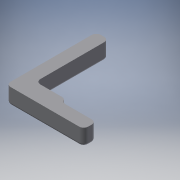
# Autodesk Inventor part: Stand_Vorne
Saved by Autodesk Inventor 2018 (Build 220112000, 112)
## iProperties
Created: 2017-12-09
Part Number: Stand_Vorne
Material: Generisch
Document SubType Name: Modeling
Designer: aXe
Density: 1 g/cm^3
Appearance: Vorgabe
Author: aXe
Autodesk Inventor part; units mm, degrees
ref_plane "YZ Plane" through (0, 0, 0) normal (1, 0, 0) x (0, 1, 0)
ref_plane "XZ Plane" through (0, 0, 0) normal (0, 1, 0) x (-1, 0, 0)
ref_plane "XY Plane" through (0, 0, 0) normal (0, 0, 1) x (1, 0, 0)
sketch "Skizze1" plane through (0, 0, 0) normal (0, 0, 1) x (1, 0, 0)
  line L0 (-2, -29) -> (-2, -31) construction
  line L1 (0, -31) -> (-2, -31) construction
  line L2 (-2, -29) -> (0, -29) construction
  line L3 (0, -31) -> (26.4999, -31) construction
  line L4 (28.4999, -31) -> (26.4999, -31) construction
  line L5 (26.4999, -29) -> (28.4999, -29) construction
  line L6 (28.4999, -31) -> (28.4999, -29) construction
  line L7 (26.4999, -29) -> (0, -29) construction
  line L8 (13, -27) -> (13, -29) construction
  line L9 (13, -27) -> (2, -27) construction
  arc A0 (0, -25) -> (2, -27) centre (2, -25) ccw construction
  arc A1 (-2, -25) -> (2, -29) centre (2, -25) ccw construction
  line L10 (-2, 0) -> (-2, -25) construction
  line L11 (0, -25) -> (0, 0) construction
  line L12 (-2, 0) -> (-2, 5) construction
  line L13 (0, 5) -> (0, 0) construction
  line L14 (0, 5) -> (-2, 5) construction
  line L15 (28.4999, -31) -> (-2, -31) construction
  line L16 (-2, -31) -> (-2, 5) construction
  line L17 (-2, 5) -> (0, 5) construction
  line L18 (0, 5) -> (0, -25) construction
  arc A2 (0, -25) -> (2, -27) centre (2, -25) ccw construction
  line L19 (2, -27) -> (13, -27) construction
  line L20 (13, -27) -> (13, -29) construction
  line L21 (13, -29) -> (28.4999, -29) construction
  line L22 (28.4999, -31) -> (28.4999, -29) construction
  line L23 (-2.25, 5.25) -> (-2.25, -31.25)
  line L24 (-2.25, -31.25) -> (28.7499, -31.25)
  line L25 (28.7499, -31.25) -> (28.7499, -28.75)
  line L26 (28.7499, -28.75) -> (13.25, -28.75)
  line L27 (13.25, -28.75) -> (13.25, -26.75)
  line L28 (13.25, -26.75) -> (2, -26.75)
  arc A3 (0.25, -25) -> (2, -26.75) centre (2, -25) ccw
  line L29 (0.25, -25) -> (0.25, 5.25)
  line L30 (0.25, 5.25) -> (-2.25, 5.25)
  line L31 (-3.75, -30.75) -> (-3.75, 4.75)
  line L32 (-1.75, 6.75) -> (-0.25, 6.75)
  line L33 (1.75, 4.75) -> (1.75, -23.25)
  arc A4 (1.75, -25) -> (2, -25.25) centre (2, -25) ccw
  line L34 (3.75, -25.25) -> (13.2859, -25.25)
  line L35 (14.75, -25.25) -> (14.75, -25.25)
  line L36 (16.75, -27.25) -> (28.2499, -27.25)
  line L37 (30.2499, -29.25) -> (30.2499, -30.75)
  line L38 (28.2499, -32.75) -> (-1.75, -32.75)
  arc A5 (28.2499, -32.75) -> (30.2499, -30.75) centre (28.2499, -30.75) ccw
  arc A6 (30.2499, -29.25) -> (28.2499, -27.25) centre (28.2499, -29.25) ccw
  arc A7 (-3.75, -30.75) -> (-1.75, -32.75) centre (-1.75, -30.75) ccw
  arc A8 (15.0179, -26.25) -> (16.75, -27.25) centre (16.75, -25.25) ccw
  arc A9 (15.0179, -26.25) -> (13.2859, -25.25) centre (13.2859, -27.25) ccw
  arc A10 (1.75, -23.25) -> (3.75, -25.25) centre (3.75, -23.25) ccw
  arc A11 (1.75, 4.75) -> (-0.25, 6.75) centre (-0.25, 4.75) ccw
  arc A12 (-1.75, 6.75) -> (-3.75, 4.75) centre (-1.75, 4.75) ccw
  dimension "d0" = 0.25
  dimension "d1" = 1.5
  dimension "d2" = 2
  dimension "d3" = 2
  constraints: 48 end point, 23 point on circle, 17 tangent, 11 centre point, 8 collinear, 6 equal radius, 3 point on line, 1 coincident, 16 other
  measures "d0" distance between parallel lines of L16 L23
  measures "d1" distance between parallel lines of L23 L31
  measures "d2" radius of A5
  measures "d3" radius of A7
extrude "Extrusion1" add sketch "Skizze1" against normal blind 5
fillet "Rundung1" radius 1 15 edges at (-3.1642, -32.1642, -5) (-3.75, -13, -5) (-3.1642, 6.1642, -5) (-1, 6.75, -5) (1.1642, 6.1642, -5) (1.75, -9.25, -5) (2.3358, -24.6642, -5) (8.5179, -25.25, -5) (14.2859, -25.5179, -5) (15.75, -26.9821, -5) (22.5, -27.25, -5) (29.6641, -27.8358, -5) (30.2499, -30, -5) (29.6641, -32.1642, -5) (13.25, -32.75, -5)
sketch "Skizze2" plane through (0, 0, 0) normal (0, 0, 1) x (1, 0, 0)
  line L0 (28.7499, -31.25) -> (-2.25, -31.25) projected
  line L1 (-2.25, -31.25) -> (-2.25, 5.25) projected
  line L2 (-2.25, 5.25) -> (0.25, 5.25) projected
  line L3 (0.25, 5.25) -> (0.25, -25) projected
  arc A0 (0.25, -25) -> (2, -26.75) centre (2, -25) ccw projected
  line L4 (2, -26.75) -> (13.25, -26.75) projected
  line L5 (13.25, -26.75) -> (13.25, -28.75) projected
  line L6 (13.25, -28.75) -> (28.7499, -28.75) projected
  line L7 (28.7499, -28.75) -> (28.7499, -31.25) projected
  line L8 (30.2499, -30.75) -> (30.2499, -29.25) projected
  arc A1 (30.2499, -29.25) -> (28.2499, -27.25) centre (28.2499, -29.25) ccw projected
  line L9 (28.2499, -27.25) -> (16.75, -27.25) projected
  arc A2 (15.0179, -26.25) -> (16.75, -27.25) centre (16.75, -25.25) ccw projected
  arc A3 (15.0179, -26.25) -> (13.2859, -25.25) centre (13.2859, -27.25) ccw projected
  line L10 (13.2859, -25.25) -> (3.75, -25.25) projected
  arc A4 (1.75, -23.25) -> (3.75, -25.25) centre (3.75, -23.25) ccw projected
  line L11 (1.75, -23.25) -> (1.75, 4.75) projected
  arc A5 (1.75, 4.75) -> (-0.25, 6.75) centre (-0.25, 4.75) ccw projected
  line L12 (-0.25, 6.75) -> (-1.75, 6.75) projected
  arc A6 (-1.75, 6.75) -> (-3.75, 4.75) centre (-1.75, 4.75) ccw projected
  line L13 (-3.75, 4.75) -> (-3.75, -30.75) projected
  arc A7 (-3.75, -30.75) -> (-1.75, -32.75) centre (-1.75, -30.75) ccw projected
  line L14 (-1.75, -32.75) -> (28.2499, -32.75) projected
  arc A8 (28.2499, -32.75) -> (30.2499, -30.75) centre (28.2499, -30.75) ccw projected
  point P0 (0, 0)
extrude "Extrusion2" add sketch "Skizze2" along normal blind 2 contours L0 L1 L2 L3 A0 L4 L5 L6 L7 | A8 L14 A7 L13 A6 L12 A5 L11 A4 L10 A3 A2 L9 A1 L8
